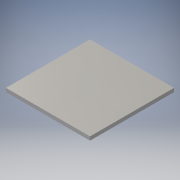
# Autodesk Inventor part: Afastador
Saved by Autodesk Inventor 2016 (Build 200138000, 138)
## iProperties
Created: 2017-04-03
Part Number: Afastador
Material: Titanium
Document SubType Name: Modeling
Designer: Marcelo
Mass: 2385.79 g
Surface Area: 1150 cm^2
Volume: 529 cm^3
Density: 4.51 g/cm^3
Appearance: Titanium
Author: Marcelo
Autodesk Inventor part; units mm, degrees
ref_plane "YZ Plane" through (0, 0, 0) normal (1, 0, 0) x (0, 1, 0)
ref_plane "XZ Plane" through (0, 0, 0) normal (0, 1, 0) x (-1, 0, 0)
ref_plane "XY Plane" through (0, 0, 0) normal (0, 0, 1) x (1, 0, 0)
sketch "Sketch1" plane through (0, 0, 0) normal (0, 0, 1) x (1, 0, 0)
  line L0 (-112.5, 115) -> (112.5, 115)
  line L1 (112.5, 115) -> (112.5, -115)
  line L2 (112.5, -115) -> (-112.5, -115)
  line L3 (-112.5, -115) -> (-112.5, 115)
  point P0 (0, 0)
  dimension "d0" = 115
  dimension "d1" = 230
  dimension "d2" = 225
  dimension "d3" = 112.5
  constraints: 8 end point, 2 parallel, 1 horizontal, 1 perpendicular
  measures "d0" distance from line of point (0, 0) L0
  measures "d1" distance of L2.end L0.start
  measures "d2" distance between parallel lines of L1 L3
  measures "d3" distance from line of point (0, 0) L3
extrude "Extrusion1" add sketch "Sketch1" along normal blind 10
equation "\"d0\" = 0.5 * d1"
equation "\"d3\" = 0.5 * d2"
body "Solid1"
